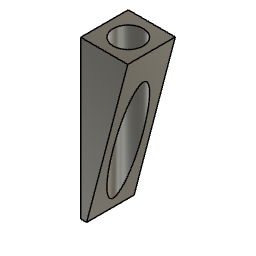
Cut+Jig (Autodesk Fusion 360 design; units mm, degrees)
Autodesk Fusion 360 part; units mm, degrees
sketch "Sketch1" plane through (0, 0, 0) normal (0, 1, 0) x (1, 0, 0)
  line L0 (0, -150) -> (0, 0)
  line L1 (0, 0) -> (37.9244, -145.1266)
  line L2 (0, 0) -> (0, 120)
  line L3 (0, 0) -> (-12.6415, 48.3755)
  dimension "d1" = 14.645
  dimension "d2" = 150
  dimension "d4" = 150
  dimension "d9" = 120
  dimension "d10" = 50
  constraint coincident L0.end L1.start
  constraint vertical L0
  constraint parallel L0 L2
  constraint parallel L1 L3
  measures "d1" angle of L0 L1
  measures "d2" distance of L0.start L0.end
  measures "d4" distance of L0.end L1.end
  measures "d9" distance of L0.end L2.end
  measures "d10" distance of L0.end L3.end
pipe "Pipe1" add diameter 58.42 wall 3.81 path "Sketch1" along L0 L2
ref_plane "WorkPlane1" through (18.9622, 0, 72.5633) normal (-0.967511, 0, 0.252829) x (0.252829, 0, 0.967511)
sketch "Sketch2" plane through (18.9622, 0, 72.5633) normal (-0.967511, 0, 0.252829) x (0.252829, 0, 0.967511)
  line L0 (271.963, -146.2875) -> (271.963, 151.3089)
  line L1 (271.963, 151.3089) -> (-728.037, 151.3089)
  line L2 (-728.037, 151.3089) -> (-728.037, -146.2875)
  line L3 (-728.037, -146.2875) -> (271.963, -146.2875)
  dimension "d18" = 1000
  constraint vertical L0
  constraint perpendicular L1 L2
  constraint perpendicular L0 L1
  constraint perpendicular L2 L3
  measures "d18" distance of L0.end L1.end
sketch "Sketch3" plane through (0, 0, 150) normal (0, 0, 1) x (-1, 0, 0)
  circle A0 centre (0, 0) radius 25.4
  circle A1 centre (0, 0) radius 29.21
  line L0 (40, -40) -> (-40, -40)
  line L1 (-40, -40) -> (-40, 40)
  line L2 (-40, 40) -> (40, 40)
  line L3 (40, 40) -> (40, -40)
  line L4 (40, -40) -> (-40, 40) construction
  line L5 (-40, -40) -> (40, 40) construction
  dimension "d19" = 80
  dimension "d20" = 80
  constraint horizontal L0
  constraint perpendicular L0 L1
  constraint parallel L0 L2
  constraint parallel L1 L3
  constraint coincident L4 A0.centre
  constraint coincident L5 A0.centre
  constraint coincident A0.centre A1.centre
  measures "d19" distance of L1.end L2.end
  measures "d20" distance of L0.end L1.end
extrude "Extrude2" add sketch "Sketch3" against normal blind 265 contours L0 L1 L2 L3
extrude "Extrude3" cut sketch "Sketch2" against normal blind 190
